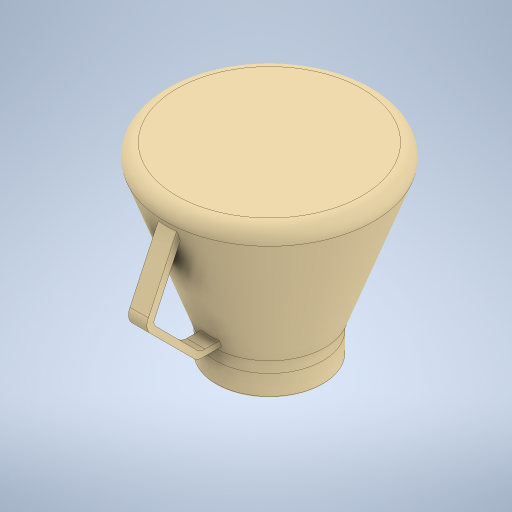
# Autodesk Inventor part: Vase
Saved by Autodesk Inventor 2024 (Build 280153000, 153)
## iProperties
Created: 2024-03-21
Part Number: Vase
Material: Stahl
Document SubType Name: Modeling
Designer: ffogue
Density: 7.85 g/cm^3
Appearance: Weizen
Author: ffogue
Autodesk Inventor part; units mm, degrees
ref_plane "YZ Plane" through (0, 0, 0) normal (1, 0, 0) x (0, 1, 0)
ref_plane "XY Plane" through (0, 0, 0) normal (0, 0, 1) x (1, 0, 0)
sketch "Skizze5" plane through (0, 0, 0) normal (0, 0, 1) x (1, 0, 0)
  circle A0 centre (0, 0) radius 180
  dimension "d8" = 360
  constraints: 1 centre point, 1 coincident
  measures "d8" diameter of A0
extrude "Extrusion2" add sketch "Skizze5" along normal blind 255
draft "Flächenverjüngung1" angle 20 pull direction (0, 0, -1) faces at (179.5615, -12.5562, 170) fixed edges at (-180, 0, 255)
fillet "Rundung1" radius 20 1 edges at (-180, 0, 255)
ref_plane "Arbeitsebene5" through (0, 0, 0) normal (0, 1, 0) x (-1, 0, 0)
sketch "Skizze7" plane through (0, 0, 0) normal (0, 1, 0) x (-1, 0, 0)
  line L0 (0, 0) -> (0, -45)
  line L1 (87.1876, 0) -> (-87.1876, 0) projected
  line L2 (87.1876, 0) -> (87.1876, -45)
  line L3 (87.1876, -45) -> (0, -45)
  dimension "d15" = 45
  constraints: 6 end point, 2 vertical, 1 perpendicular
  measures "d15" distance of L0.start L0.end
revolve "Umdrehung1" add sketch "Skizze7" angle 360 about axis through (0, 0, 0) along (0, 0, -1)
fillet "Rundung2" radius 60 2 edges at (0, 87.1876, 0) (0, -87.1876, 0)
shell "Wandung1" thickness 8 removed faces 1 at (6.467, -28.3339, -45)
sketch "Skizze8" plane through (0, 0, 0) normal (1, 0, 0) x (0, 1, 0)
  line L0 (-90.806, 9.9416) -> (-170.2309, 228.1596) projected
  line L1 (-83.2885, 12.6778) -> (-162.7134, 230.8958) projected
  line L2 (-83.2885, 12.6778) -> (-162.7134, 230.8958) projected
  line L3 (-87.1876, -10.5796) -> (-87.1876, -45) projected
  line L4 (-87.1876, -10.5796) -> (-87.1876, -45) projected
  line L5 (79.1876, -45) -> (-79.1876, -45) projected
  line L6 (-79.1876, -10.5796) -> (-79.1876, -45) projected
  line L7 (-79.1876, -10.5796) -> (-79.1876, -45) projected
  arc A0 (-79.1876, -10.5796) -> (-83.2885, 12.6778) centre (-147.1876, -10.5796) ccw projected
  arc A1 (-79.1876, -10.5796) -> (-83.2885, 12.6778) centre (-147.1876, -10.5796) ccw projected
  line L8 (-87.1876, -45) -> (87.1876, -45) projected
  arc A2 (-87.1876, -10.5796) -> (-90.806, 9.9416) centre (-147.1876, -10.5796) ccw projected
  arc A3 (-87.1876, -10.5796) -> (-90.806, 9.9416) centre (-147.1876, -10.5796) ccw projected
  arc A4 (-151.437, 255) -> (-170.2309, 228.1596) centre (-151.437, 235) ccw projected
  arc A5 (-151.437, 255) -> (-170.2309, 228.1596) centre (-151.437, 235) ccw projected
  line L9 (-151.437, 255) -> (151.437, 255) projected
  arc A6 (170.2309, 228.1596) -> (151.437, 255) centre (151.437, 235) ccw projected
  line L10 (90.806, 9.9416) -> (170.2309, 228.1596) projected
  line L11 (87.1876, -10.5796) -> (87.1876, -45) projected
  arc A7 (90.806, 9.9416) -> (87.1876, -10.5796) centre (147.1876, -10.5796) ccw projected
  line L12 (-83.2885, 12.6778) -> (83.2885, 12.6778) projected
  line L13 (-96.2868, 25) -> (-126.2868, 25) construction
  arc A8 (-131.0068, 25.5649) -> (-126.2868, 25) centre (-126.2868, 45) ccw construction
  line L14 (-131.0068, 25.5649) -> (-201.7175, 96.2756) construction
  arc A9 (-205.7015, 118.8701) -> (-201.7175, 96.2756) centre (-187.5753, 110.4177) ccw construction
  line L15 (-205.7015, 118.8701) -> (-163.4397, 209.5009) construction
  line L16 (-94.467, 20) -> (-124.467, 20)
  arc A10 (-138.6091, 25.8579) -> (-124.467, 20) centre (-124.467, 40) ccw
  line L17 (-138.6091, 25.8579) -> (-209.3198, 96.5685)
  line L18 (-98.1067, 30) -> (-120.0865, 30)
  arc A11 (-134.2287, 35.8579) -> (-120.0865, 30) centre (-120.0865, 50) ccw
  line L19 (-134.2287, 35.8579) -> (-200.6967, 102.3259)
  arc A12 (-202.6887, 113.6232) -> (-200.6967, 102.3259) centre (-193.6256, 109.397) ccw
  line L20 (-202.6887, 113.6232) -> (-161.0464, 202.9254)
  arc A13 (-212.7349, 120.2889) -> (-209.3198, 96.5685) centre (-195.1777, 110.7107) ccw
  line L21 (-212.7349, 120.2889) -> (-166.813, 218.7689)
  line L22 (-94.467, 20) -> (-93.467, 20)
  line L23 (-93.467, 20) -> (-97.1067, 30)
  line L24 (-97.1067, 30) -> (-98.1067, 30)
  point P0 (0, 0)
  point P1 (-111.2868, 25)
  point P2 (-109.467, 20)
  dimension "d22" = 70
  dimension "d23" = 20
  dimension "d24" = 100
  dimension "d25" = 20
  dimension "d26" = 110
  dimension "d27" = 100
  dimension "d28" = 135
  dimension "d29" = 30
  dimension "d33" = 5
  dimension "d35" = 5
  dimension "d36" = 5
  dimension "d37" = 20
  dimension "d38" = 10
  dimension "d39" = 94
  dimension "d40" = 20
  dimension "d41" = 6.9741
  dimension "d44" = 1
  constraints: 24 end point, 12 point on circle, 10 tangent, 7 parallel, 6 centre point, 4 horizontal, 2 midpoint, 1 equal radius, 8 other
  measures "d22" distance from line of point (-111.287, 25) L5
  measures "d23" radius of A8
  measures "d24" distance of L14.start L14.end
  measures "d25" radius of A9
  measures "d26" angle of L15 L14
  measures "d27" distance of L15.start L15.end
  measures "d28" angle of L14 L13
  measures "d29" distance of L13.start L13.end
  measures "d33" vertical distance of point (-111.287, 25) point (-109.467, 20)
  measures "d35" distance between parallel lines of L18 L13
  measures "d36" distance between parallel lines of L14 L19
  measures "d37" radius of A11
  measures "d38" radius of A12
  measures "d39" distance of L19.start L19.end
  measures "d40" radius of A13
  measures "d41" distance between parallel lines of L21 L15
  measures "d44" distance of L16.start L22.end
extrude "Extrusion4" add sketch "Skizze8" along normal mid plane 30 fills toward (-189.7286, 169.5078) open curves L21 A13 L17 A10 L16 L22 L23 L24 L18 A11 L19 A12 L20
fillet "Rundung3" radius 2 1 edges at (87.1876, 0, -45)
equation "\"d35\" = d33"
equation "\"d36\" = d33"
equation "\"d37\" = d23"
